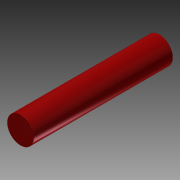
# Autodesk Inventor part: 知能ロボコンばね受け
Saved by Autodesk Inventor 2013 (Build 170138000, 138)
## iProperties
Created: 2014-05-12
Part Number: 知能ロボコンばね受け
Material: 一般
Document SubType Name: Modeling
Designer: horumo136
Density: 1 g/cm^3
Author: horumo136
Autodesk Inventor part; units mm, degrees
ref_plane "YZ Plane" through (0, 0, 0) normal (1, 0, 0) x (0, 1, 0)
ref_plane "XZ Plane" through (0, 0, 0) normal (0, 1, 0) x (-1, 0, 0)
ref_plane "XY Plane" through (0, 0, 0) normal (0, 0, 1) x (1, 0, 0)
sketch "スケッチ1" plane through (0, 0, 0) normal (0, 1, 0) x (-1, 0, 0)
  circle A0 centre (0, 0) radius 7
  dimension "d0" = 14
  constraints: 1 centre point, 1 coincident
  measures "d0" diameter of A0
extrude "押し出し1" add sketch "スケッチ1" along normal blind 70
sketch "スケッチ2" plane through (0, 70, 0) normal (0, 1, 0) x (1, 0, 0)
  circle A0 centre (0, 0) radius 7 projected
sketch "スケッチ3" plane through (0, 70, 0) normal (0, 1, 0) x (1, 0, 0)
  circle A0 centre (0, 0) radius 7 projected
  circle A1 centre (0, 0) radius 27.5
  dimension "d3" = 55
  constraints: 1 centre point, 1 coincident
  measures "d3" diameter of A1
extrude "押し出し2" add sketch "スケッチ3" along normal blind 3
extrude "押し出し3" add sketch "スケッチ2" along normal blind 3
sketch "スケッチ4" plane through (0, 73, 0) normal (0, 1, 0) x (1, 0, 0)
  circle A0 centre (0, 0) radius 27.5 projected
  circle A1 centre (0, 0) radius 25
  line L0 (0, 0) -> (17.6777, 17.6777)
  line L1 (0, 0) -> (25, 0) construction
  circle A2 centre (17.6777, 17.6777) radius 1.5
  circle A3 centre (-17.6777, 17.6777) radius 1.5
  circle A4 centre (-17.6777, -17.6777) radius 1.5
  circle A5 centre (17.6777, -17.6777) radius 1.5
  dimension "d8" = 50
  dimension "d9" = 45
  dimension "d10" = 3
  dimension "d13" = 360
  constraints: 4 centre point, 4 end point, 3 coincident, 1 equal length, 1 horizontal, 12 other
  measures "d9" angle of L1 L0
  measures "d10" diameter of A2
hole "穴1" at (0, 73, 0) at (-17.6777, 73, -17.6777) at (17.6777, 73, -17.6777) at (17.6777, 73, 17.6777) at (-17.6777, 73, 17.6777) direction (0, -1, 0) diameter 3 depth 8 tip angle 118
sketch "スケッチ6" plane through (0, 70, 0) normal (0, -1, 0) x (1, 0, 0)
  circle A0 centre (17.6777, 17.6777) radius 1.5 projected
  circle A1 centre (-17.6777, -17.6777) radius 1.5 projected
  circle A2 centre (17.6777, -17.6777) radius 1.5 projected
  circle A3 centre (-17.6777, 17.6777) radius 1.5 projected
  circle A4 centre (0, 0) radius 7 projected
  circle A5 centre (0, 0) radius 27.5 projected
extrude "押し出し5" cut sketch "スケッチ6" against normal blind 3
sketch "スケッチ7" plane through (0, 73, 0) normal (0, 1, 0) x (1, 0, 0)
  circle A0 centre (0, 0) radius 1.5 projected
  circle A1 centre (0, 0) radius 1.5
  constraints: 1 centre point, 1 coincident, 1 concentric
extrude "押し出し6" add sketch "スケッチ7" against normal blind 73
